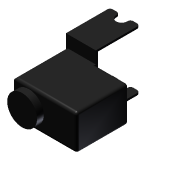
# Autodesk Inventor part: Wrist
Saved by Autodesk Inventor 2012 (Build 160160000, 160)
## iProperties
Created: 2013-02-21
Part Number: Wrist
Material: Default
Document SubType Name: Modeling
Designer: Andrew
Density: 1 g/cm^3
Author: Andrew
Autodesk Inventor part; units mm, degrees
ref_plane "YZ Plane" through (0, 0, 0) normal (1, 0, 0) x (0, 1, 0)
ref_plane "XZ Plane" through (0, 0, 0) normal (0, 1, 0) x (-1, 0, 0)
ref_plane "XY Plane" through (0, 0, 0) normal (0, 0, 1) x (1, 0, 0)
sketch "Sketch1" plane through (0, 0, 0) normal (0, 0, 1) x (1, 0, 0)
  line L0 (5.75, 38.85) -> (2.7639, 38.85)
  arc A0 (2.7639, 38.85) -> (0.767, 36.9611) centre (2.7639, 36.85) ccw
  arc A1 (0.767, 36.9611) -> (0.75, 36.35) centre (11.75, 36.35) ccw
  line L1 (0.75, 7.85) -> (0.75, 36.35)
  line L2 (22.75, 7.85) -> (0.75, 7.85)
  line L3 (22.75, 7.85) -> (22.75, 36.35)
  arc A2 (22.75, 36.35) -> (22.733, 36.9611) centre (11.75, 36.35) ccw
  arc A3 (22.733, 36.9611) -> (20.7361, 38.85) centre (20.7361, 36.85) ccw
  line L4 (20.7361, 38.85) -> (17.75, 38.85)
  arc A4 (17.75, 38.85) -> (15.75, 36.85) centre (17.75, 36.85) ccw
  line L5 (15.75, 36.85) -> (15.75, 36.35)
  arc A5 (7.75, 36.35) -> (15.75, 36.35) centre (11.75, 36.35) ccw
  line L6 (7.75, 36.85) -> (7.75, 36.35)
  arc A6 (7.75, 36.85) -> (5.75, 38.85) centre (5.75, 36.85) ccw
  line L7 (6.75, 13.35) -> (6.75, 15.35)
  arc A7 (7.75, 16.35) -> (6.75, 15.35) centre (7.75, 15.35) ccw
  line L8 (7.75, 16.35) -> (15.75, 16.35)
  arc A8 (16.75, 15.35) -> (15.75, 16.35) centre (15.75, 15.35) ccw
  line L9 (16.75, 15.35) -> (16.75, 13.35)
  arc A9 (15.75, 12.35) -> (16.75, 13.35) centre (15.75, 13.35) ccw
  line L10 (15.75, 12.35) -> (7.75, 12.35)
  arc A10 (6.75, 13.35) -> (7.75, 12.35) centre (7.75, 13.35) ccw
  line L11 (6.75, 21.35) -> (6.75, 23.35)
  arc A11 (7.75, 24.35) -> (6.75, 23.35) centre (7.75, 23.35) ccw
  line L12 (7.75, 24.35) -> (15.75, 24.35)
  arc A12 (16.75, 23.35) -> (15.75, 24.35) centre (15.75, 23.35) ccw
  line L13 (16.75, 23.35) -> (16.75, 21.35)
  arc A13 (15.75, 20.35) -> (16.75, 21.35) centre (15.75, 21.35) ccw
  line L14 (15.75, 20.35) -> (7.75, 20.35)
  arc A14 (6.75, 21.35) -> (7.75, 20.35) centre (7.75, 21.35) ccw
  circle A15 centre (3.75, 18.35) radius 1.1
  circle A16 centre (19.75, 18.35) radius 1.1
  circle A17 centre (19.75, 36.35) radius 1
  circle A18 centre (17.4069, 30.6931) radius 1
  circle A19 centre (11.75, 28.35) radius 1
  circle A20 centre (6.0931, 30.6931) radius 1
  circle A21 centre (3.75, 36.35) radius 1
  line L15 (11.75, 7.85) -> (11.75, 6.35)
  line L16 (22.75, 7.85) -> (22.75, 6.35)
  line L17 (22.75, 6.35) -> (0.75, 6.35)
  line L18 (0.75, 6.35) -> (0.75, 7.85)
  line L19 (22.75, 6.35) -> (47, 6.35)
  line L20 (11.75, 6.35) -> (11.75, -37)
  line L21 (11.75, -37) -> (22.75, -37)
  line L22 (11.75, -37) -> (0.75, -37)
  line L23 (0.75, -37) -> (0.75, -32)
  line L24 (0.75, -32) -> (22.75, -32)
  line L25 (22.75, -32) -> (22.75, -37)
  line L26 (0.75, -32) -> (0.75, 6.35)
  line L27 (22.75, -32) -> (47, -32)
  line L28 (47, -32) -> (47, 6.35)
  dimension "d0" = 24.25
  dimension "d1" = 43.35
  dimension "d2" = 11
  dimension "d3" = 11
  dimension "d4" = 5
  constraints: 28 end point, 7 perpendicular, 4 parallel, 2 collinear, 1 midpoint
  measures "d0" distance of L16.end L19.end
  measures "d1" distance of L15.end L20.end
  measures "d2" distance of L20.end L21.end
  measures "d3" distance of L20.end L22.end
  measures "d4" distance of L22.end L23.end
extrude "Extrusion1" add sketch "Sketch1" along normal mid plane 26 contours L17 L20 L24 L26 | L17 L19 L28 L27 L24 L20
sketch "Sketch2" plane through (0.75, -32, 13) normal (0, -1, 0) x (1, 0, 0)
  circle A0 centre (11, -13) radius 11
  point P0 (-0.75, -13)
  dimension "d8" = 22
  constraints: 1 centre point
  measures "d8" diameter of A0
extrude "Extrusion2" add sketch "Sketch2" along normal blind 5
sketch "Sketch3" plane through (0.75, 6.35, 13) normal (0, 1, 0) x (1, 0, 0)
  line L0 (0, 26) -> (0, 0) projected
  line L1 (0, 13) -> (0, -7.5)
  line L2 (0, -7.5) -> (22, -7.5)
  line L3 (22, -7.5) -> (22, 33.5)
  line L4 (22, 33.5) -> (0, 33.5)
  line L5 (0, 33.5) -> (0, 13)
  line L6 (0, 33.5) -> (0, 35)
  line L7 (0, 35) -> (22, 35)
  line L8 (22, 35) -> (22, 33.5)
  line L9 (22, -7.5) -> (22, -9)
  line L10 (22, -9) -> (0, -9)
  line L11 (0, -9) -> (0, -7.5)
  point P0 (-0.75, 13)
  dimension "d13" = 20.5
  dimension "d14" = 22
  dimension "d15" = 41
  dimension "d16" = 1.5
  dimension "d17" = 1.5
  constraints: 22 end point, 4 perpendicular, 3 collinear, 3 parallel, 1 midpoint, 1 point on line
  measures "d13" distance of L1.start L1.end
  measures "d14" distance of L1.end L2.end
  measures "d15" distance of L2.end L3.end
  measures "d16" distance of L4.end L6.end
  measures "d17" distance of L2.end L9.end
extrude "Extrusion3" add sketch "Sketch3" along normal blind 1.5
sketch "Sketch4" plane through (0.75, 7.85, 13) normal (0, 1, 0) x (1, 0, 0)
  line L0 (0, -9) -> (0, 35) projected
  line L1 (22, -9) -> (0, -9) projected
  line L2 (22, 35) -> (22, -9) projected
  line L3 (0, 35) -> (22, 35) projected
  line L4 (22, -9) -> (22, -7.5)
  line L5 (22, -7.5) -> (0, -7.5)
  line L6 (0, 35) -> (0, 33.5)
  line L7 (0, 33.5) -> (22, 33.5)
  line L8 (22, 33.5) -> (22, 35)
  line L9 (22, 35) -> (0, 35)
  line L10 (21.4157, -9) -> (0, -9)
  line L11 (0, -7.5) -> (0, -9)
  point P0 (-0.75, 13)
  dimension "d20" = 1.5
  dimension "d21" = 1.5
  constraints: 16 end point, 5 point on line, 3 perpendicular, 2 collinear, 1 parallel
  measures "d20" distance of L1.start L4.end
  measures "d21" distance of L0.end L6.end
extrude "Extrusion4" add sketch "Sketch4" along normal blind 35 contours L0 L5 L2 L1 | L0 L3 L2 L7
sketch "Sketch5" plane through (0.75, 7.85, -20.5) normal (0, 0, 1) x (1, 0, 0)
  line L0 (22, 35) -> (0, 35) projected
  line L1 (0, 0) -> (0, 35) projected
  line L2 (22, 0) -> (22, 35) projected
  line L3 (5, 31) -> (2.0139, 31) projected
  arc A0 (2.0139, 31) -> (0.017, 29.1111) centre (2.0139, 29) ccw projected
  arc A1 (0.017, 29.1111) -> (0, 28.5) centre (11, 28.5) ccw projected
  arc A2 (7, 28.5) -> (15, 28.5) centre (11, 28.5) ccw projected
  arc A3 (7, 29) -> (5, 31) centre (5, 29) ccw projected
  line L4 (7, 29) -> (7, 28.5) projected
  line L5 (15, 29) -> (15, 28.5) projected
  arc A4 (17, 31) -> (15, 29) centre (17, 29) ccw projected
  line L6 (19.9861, 31) -> (17, 31) projected
  arc A5 (21.983, 29.1111) -> (19.9861, 31) centre (19.9861, 29) ccw projected
  arc A6 (22, 28.5) -> (21.983, 29.1111) centre (11, 28.5) ccw projected
  point P0 (-0.75, -7.85)
extrude "Extrusion5" cut sketch "Sketch5" along normal through all both and the other way through all
fillet "Fillet1" radius 2 10 edges at (47, -12.825, -13) (47, -12.825, 13) (47, -32, 0) (23.875, -32, 13) (23.875, -32, -13) (34.875, 6.35, -13) (34.875, 6.35, 13) (0.75, -12.825, -13) (0.75, -12.825, 13) (47, 6.35, 0)
body "Solid1"
